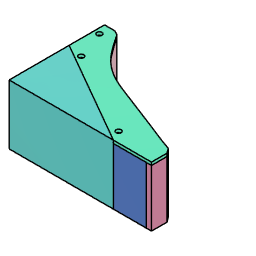
Version-1-reposabajo (Autodesk Fusion 360 archive; units mm, degrees)
design "Gomas bajo"
Autodesk Fusion 360 part; units mm, degrees
note: some values were not read from the file. Chosen so that the rebuilt part matches the saved one: which bodies a step acts on. Set by a fixed rule: which sketch regions a step uses.
sketch "Boceto1" plane through (0, 0, 0) normal (0, 1, 0) x (1, 0, 0)
  line L0 (0, 0) -> (381, 0)
  line L1 (0, 0) -> (0, 64.9)
  line L2 (381, 0) -> (381, 54.6)
  line L3 (381, 54.6) -> (327.1, 0)
  line L4 (0, 64.9) -> (168.7, 0)
  line L5 (0, 0) -> (0, 109.3)
  line L6 (0, 109.3) -> (62.7, 0)
  line L7 (168.7, 0) -> (168.7, 23.3)
  line L8 (168.7, 23.3) -> (326.4, 23.3)
  line L9 (326.4, 23.3) -> (326.4, 0)
  line L10 (0, 0) -> (0, -78.7)
  line L11 (0, -78.7) -> (-56.8, -78.7)
  line L12 (-56.8, -78.7) -> (-56.8, 0)
  line L13 (-56.8, 0) -> (0, 0)
  line L14 (0, 109.3) -> (168.7, 0)
  line L15 (32.6827, 52.3267) -> (381, 54.6)
  circle A0 centre (0, 64.9) radius 22.093
  line L16 (19.1638, 75.8933) -> (0, 64.9)
  arc A1 (19.1638, 75.8933) -> (58.0399, 42.5717) centre (85.4981, 113.946) ccw
  line L17 (104.1577, -30) -> (104.1577, 0)
  arc A2 (145.6154, 0) -> (62.7, 0) centre (104.1577, -30) ccw
  dimension "d1" = 381
  dimension "d2" = 64.9
  dimension "d3" = 54.6
  dimension "d4" = 53.9
  dimension "d5" = 168.7
  dimension "d6" = 109.3
  dimension "d7" = 62.7
  dimension "d8" = 23.3
  dimension "d9" = 157.7
  dimension "d10" = 78.7
  dimension "d11" = 56.8
  dimension "d14" = 30
  constraint coincident L0.start L1.start
  constraint horizontal L0
  constraint perpendicular L0 L1
  constraint perpendicular L0 L2
  constraint coincident L0 L3.end
  constraint coincident L0 L4.end
  constraint perpendicular L0 L5
  constraint coincident L0 L6.end
  constraint perpendicular L0 L7
  constraint perpendicular L7 L8
  constraint coincident L0 L9.end
  constraint perpendicular L0 L9
  constraint perpendicular L0 L10
  constraint perpendicular L10 L11
  constraint perpendicular L11 L12
  constraint perpendicular L10 L13
  constraint coincident L6 L15.start
  constraint coincident L4 L15.start
  constraint coincident L1.end L4.start
  constraint tangent L6 A0
  constraint tangent L6 A1
  constraint tangent L4 A1
  constraint coincident L6 L16.start
  constraint coincident A0 L16.start
  constraint perpendicular L6 L16
  constraint coincident L4 A1.end
  constraint tangent L4 A2
  constraint coincident L17.start A2.centre
  constraint coincident L0 L17.end
  constraint perpendicular L0 L17
  constraint coincident L0 A2.start
  measures "d1" distance of L0.start L0.end
  measures "d2" distance of L0.start L1.end
  measures "d3" distance of L0.end L2.end
  measures "d4" distance of L0.end L3.end
  measures "d5" distance of L0.start L4.end
  measures "d6" distance of L0.start L5.end
  measures "d7" distance of L0.start L6.end
  measures "d8" distance of L4.end L7.end
  measures "d9" distance of L7.end L8.end
  measures "d10" distance of L0.start L10.end
  measures "d11" distance of L10.end L11.end
  measures "d14" distance of L17.start L17.end
extrude "Extruir1" add sketch "Boceto1" along normal blind 120 contours L0 L1 L4 L5 L6 A0 | L10 L11 L12 L13 | L0 A2 | L4 L6 A2 | L1 L4 L5 A0 | L4 L15 A1 | L4 L6 A0 | L6 L15 A1 | L4 A0 L16 | L5 A0 L16 | L0 L7 L8 L9 | L0 L2 L3 makes body 3 at (48.5385, 80, 0) makes body 3 at (0, 40, 26.2333) makes body 2 at (363.0333, 40, -36.4) makes body 1 at (221.2667, 40, -23.3)
sketch "Boceto2" plane through (0, 120, 0) normal (0, 1, 0) x (-1, 0, 0)
  line L0 (0, 0) -> (-145.6154, 0)
  arc A0 (-145.6154, 0) -> (-122.5313, -17.7614) centre (-104.1577, 30) ccw
  line L1 (-122.5313, -17.7614) -> (-58.0399, -42.5717)
  arc A1 (-19.1638, -75.8933) -> (-58.0399, -42.5717) centre (-85.4981, -113.946) ccw
  arc A2 (-19.1638, -75.8933) -> (0, -86.993) centre (0, -64.9) ccw
  line L2 (0, -86.993) -> (0, 0)
  arc A3 (-137.514, 5.8624) -> (-118.9408, -8.4282) centre (-104.1577, 30) ccw
  line L3 (-118.9408, -8.4282) -> (-54.4494, -33.2385)
  arc A4 (-10.4896, -70.9174) -> (-54.4494, -33.2385) centre (-85.4981, -113.946) ccw
  arc A5 (-10.4896, -70.9174) -> (0, -76.993) centre (0, -64.9) ccw
  line L4 (-10, -84.6003) -> (-10, -10)
  line L5 (-10, -10) -> (-136.0754, -10)
  line L6 (-10.4896, -70.9174) -> (-85.4981, -113.946)
  line L7 (-85.4981, -113.946) -> (-54.4494, -33.2385)
  arc A6 (-143.9951, 1.1725) -> (-121.8132, -15.8948) centre (-104.1577, 30) ccw
  line L8 (-121.8132, -15.8948) -> (-57.3218, -40.705)
  arc A7 (-17.4289, -74.8981) -> (-57.3218, -40.705) centre (-85.4981, -113.946) ccw
  arc A8 (-17.4289, -74.8981) -> (0, -84.993) centre (0, -64.9) ccw
  arc A9 (-14.7871, -64.1697) -> (-4.4377, -76.1494) centre (-10.4896, -70.9174) ccw
  arc A10 (-24.2647, -52.887) -> (-14.0734, -65.1993) centre (-18.884, -58.8072) ccw
  arc A11 (-35.5202, -43.3773) -> (-23.3866, -53.7805) centre (-29.2125, -48.298) ccw
  arc A12 (-48.2269, -35.9166) -> (-34.5032, -44.1087) centre (-41.1754, -39.6949) ccw
  arc A13 (-61.8917, -30.3754) -> (-47.1004, -36.4648) centre (-54.4252, -33.2478) ccw
  arc A14 (-75.8914, -24.9896) -> (-60.9584, -30.7344) centre (-68.4249, -27.862) ccw
  arc A15 (-89.8912, -19.6038) -> (-74.9581, -25.3486) centre (-82.4247, -22.4762) ccw
  arc A16 (-103.891, -14.218) -> (-88.9579, -19.9628) centre (-96.4244, -17.0904) ccw
  arc A17 (-117.8907, -8.8322) -> (-102.9576, -14.577) centre (-110.4242, -11.7046) ccw
  arc A18 (-130.436, -1.6973) -> (-117.3466, -9.0415) centre (-124.4239, -6.3188) ccw
  arc A19 (-18.1953, -68.7673) -> (-19.5747, -66.7773) centre (-19.7105, -68.3445) ccw
  arc A20 (-26.8428, -57.9966) -> (-28.54, -56.2697) centre (-28.4078, -57.8372) ccw
  arc A21 (-37.1934, -48.8504) -> (-39.1592, -47.4367) centre (-38.7627, -48.959) ccw
  arc A22 (-48.9466, -41.5943) -> (-51.1238, -40.5349) centre (-50.4747, -41.9678) ccw
  arc A23 (-62.0016, -35.8165) -> (-64.5236, -34.8462) centre (-63.6663, -36.3809) ccw
  arc A24 (-76.0013, -30.4307) -> (-78.5233, -29.4604) centre (-77.6661, -30.9951) ccw
  arc A25 (-90.0011, -25.0449) -> (-92.5231, -24.0746) centre (-91.6658, -25.6093) ccw
  arc A26 (-104.0008, -19.6591) -> (-106.5228, -18.6888) centre (-105.6656, -20.2235) ccw
  arc A27 (-118.0703, -14.0576) -> (-120.7709, -12.9639) centre (-119.8658, -14.6102) ccw
  line L9 (-381, -54.6) -> (-327.1, 0)
  line L10 (-327.1, 0) -> (-381, 0)
  line L11 (-381, 0) -> (-381, -54.6)
  line L12 (-168.7, 0) -> (-326.4, 0)
  arc A28 (-288.7387, 0) -> (-354.05, -27.3) centre (-288.7387, -91.774) ccw
  line L13 (-354.05, -27.3) -> (-381, -54.6)
  arc A29 (-288.7387, 3) -> (-356.185, -25.1924) centre (-288.7387, -91.774) ccw
  line L14 (-356.185, -25.1924) -> (-383.135, -52.4924)
  arc A30 (-288.7387, 10) -> (-361.1665, -20.2747) centre (-288.7387, -91.774) ccw
  line L15 (-361.1665, -20.2747) -> (-388.1165, -47.5747)
  line L16 (-288.7387, -91.774) -> (-288.7387, 10)
  line L17 (-361.1665, -20.2747) -> (-288.7387, -91.774)
  arc A31 (-375.2171, -34.5078) -> (-365.3817, -24.5446) centre (-370.2994, -29.5262) ccw
  arc A32 (-381, -31.9555) -> (-374.5146, -33.7961) centre (-379.4323, -38.7777) ccw
  arc A33 (-366.0843, -25.2563) -> (-356.0804, -15.4652) centre (-361.1665, -20.2747) ccw
  arc A34 (-356.5009, -15.8383) -> (-345.4457, -7.2621) centre (-351.1209, -11.36) ccw
  arc A35 (-345.9117, -7.5766) -> (-333.8234, -0.5309) centre (-339.9888, -3.8458) ccw
  arc A36 (-334.3267, -0.7813) -> (-321.416, 4.6114) centre (-327.9641, 2.1372) ccw
  arc A37 (-330.9794, -4.1801) -> (-333.0783, -6.056) centre (-331.6366, -5.5569) ccw
  arc A38 (-342.146, -10.5051) -> (-344.138, -11.8497) centre (-342.6161, -11.9565) ccw
  arc A39 (-352.3824, -18.2454) -> (-354.18, -19.8407) centre (-352.6573, -19.7461) ccw
  arc A40 (-361.7084, -27.2537) -> (-363.328, -28.8943) centre (-361.8252, -28.7581) ccw
  arc A41 (-370.8413, -36.5052) -> (-372.4609, -38.1458) centre (-370.9581, -38.0096) ccw
  line L18 (-332.7328, 0) -> (-321.2984, 0)
  arc A42 (-133.4633, 8.7936) -> (-117.1456, -3.7616) centre (-104.1577, 30) ccw
  line L19 (-117.1456, -3.7616) -> (-52.6541, -28.5719)
  arc A43 (-6.1526, -68.4294) -> (-52.6541, -28.5719) centre (-85.4981, -113.946) ccw
  arc A44 (-6.1526, -68.4294) -> (0, -71.993) centre (0, -64.9) ccw
  line L20 (-321.2984, 0) -> (-321.2984, 10)
  line L21 (-341, 10) -> (-321.2984, 10)
  line L22 (-341, 10) -> (-381, -30)
  line L23 (-381, 0) -> (-386, 0)
  line L24 (-386, 0) -> (-386, -54.6)
  line L25 (-386, -54.6) -> (-381, -54.6)
  point P0 (-10.4896, -70.9174)
  point P1 (-18.884, -58.8072)
  point P2 (-29.2125, -48.298)
  point P3 (-41.1754, -39.6949)
  point P4 (-54.4252, -33.2478)
  point P5 (-68.4249, -27.862)
  point P6 (-82.4247, -22.4762)
  point P7 (-96.4244, -17.0904)
  point P8 (-110.4242, -11.7046)
  point P9 (-124.4239, -6.3188)
  point P10 (-351.1209, -11.36)
  point P11 (-339.9888, -3.8458)
  point P12 (-327.9641, 2.1372)
  point P13 (-315.2564, 6.4846)
  point P14 (-302.0868, 9.1209)
  point P15 (-288.6848, 10)
  point P16 (-370.2994, -29.5262)
  point P17 (-379.4323, -38.7777)
  dimension "d15" = -10
  dimension "d19" = 39.117
  dimension "d21" = 39.1
  dimension "d24" = -15
  dimension "d25" = 0
  dimension "d26" = -2
  dimension "d27" = 3
  dimension "d28" = 10
  dimension "d30" = -45.4
  dimension "d33" = 13
  dimension "d34" = 0
  dimension "d37" = -15
  dimension "d38" = 10
  dimension "d39" = 45
  dimension "d40" = 30
  dimension "d41" = 5
  constraint coincident A2 L4.start
  constraint coincident A0 L5.end
  constraint coincident P0 A4.start
  constraint coincident A1.centre A4.centre
  constraint coincident A7.start A9
  constraint coincident P1 A10.centre
  constraint tangent A7 A10
  constraint coincident P2 A11.centre
  constraint tangent A7 A11
  constraint coincident P3 A12.centre
  constraint tangent A7 A12
  constraint coincident P4 A13.centre
  constraint coincident L8.end A13
  constraint coincident P5 A14.centre
  constraint tangent L8 A14
  constraint coincident P6 A15.centre
  constraint tangent L8 A15
  constraint coincident P7 A16.centre
  constraint tangent L8 A16
  constraint coincident P8 A17.centre
  constraint tangent L8 A17
  constraint coincident P9 A18.centre
  constraint tangent A6 A18
  constraint coincident A5 A9.end
  constraint coincident A4 A10.end
  constraint coincident A4 A9.start
  constraint coincident A4 A10.start
  constraint coincident A4 A11.end
  constraint coincident A4 A12.end
  constraint coincident A4 A11.start
  constraint coincident A4 A12.start
  constraint coincident A4 A13.end
  constraint coincident L3 A14.end
  constraint coincident L3 A13.start
  constraint coincident L3 A15.end
  constraint coincident L3 A14.start
  constraint coincident L3 A15.start
  constraint coincident L3 A16.end
  constraint coincident L3 A17.end
  constraint coincident L3 A16.start
  constraint coincident L3 A18.end
  constraint coincident L3 A17.start
  constraint coincident A3 A18.start
  constraint tangent A7 A19
  constraint tangent A10 A19
  constraint tangent A9 A19
  constraint tangent A10 A20
  constraint tangent A11 A20
  constraint tangent A7 A20
  constraint tangent A7 A21
  constraint tangent A11 A21
  constraint tangent A12 A21
  constraint tangent A7 A22
  constraint tangent A13 A22
  constraint tangent A12 A22
  constraint tangent L8 A23
  constraint tangent A13 A23
  constraint tangent A14 A23
  constraint tangent A14 A24
  constraint tangent L8 A24
  constraint tangent A15 A24
  constraint tangent A15 A25
  constraint tangent L8 A25
  constraint tangent A16 A25
  constraint tangent A16 A26
  constraint tangent A17 A26
  constraint tangent L8 A26
  constraint tangent A17 A27
  constraint tangent A18 A27
  constraint tangent A6 A27
  constraint coincident A9 A19.start
  constraint coincident A10 A19.end
  constraint coincident A10 A20.start
  constraint coincident A11 A20.end
  constraint coincident A11 A21.start
  constraint coincident A12 A21.end
  constraint coincident A13 A22.end
  constraint coincident A12 A22.start
  constraint coincident A13 A23.start
  constraint coincident A14 A23.end
  constraint coincident A14 A24.start
  constraint coincident A15 A24.end
  constraint coincident A15 A25.start
  constraint coincident A16 A25.end
  constraint coincident A16 A26.start
  constraint coincident A17 A26.end
  constraint coincident A18 A27.end
  constraint coincident A17 A27.start
  constraint tangent L9 A28
  constraint tangent L12 A28
  constraint midpoint L9 A28.end
  constraint coincident L12 A28.start
  constraint coincident L9.start L11.end
  constraint coincident A28.centre A29.centre
  constraint perpendicular L12 L16
  constraint coincident P12 A36.centre
  constraint coincident P11 A35.centre
  constraint coincident P10 A34.centre
  constraint coincident A30.end L15.start
  constraint coincident P16 A31.centre
  constraint coincident P17 A32.centre
  constraint tangent A29 A36
  constraint tangent A29 A35
  constraint tangent A29 A34
  constraint tangent A29 A33
  constraint tangent L14 A31
  constraint tangent L14 A32
  constraint tangent A36 A37
  constraint tangent A35 A37
  constraint tangent A29 A37
  constraint tangent A34 A38
  constraint tangent A35 A38
  constraint tangent A29 A38
  constraint tangent A29 A39
  constraint tangent A34 A39
  constraint tangent A33 A39
  constraint tangent L14 A40
  constraint tangent A33 A40
  constraint tangent A31 A40
  constraint tangent L14 A41
  constraint tangent A31 A41
  constraint tangent A32 A41
  constraint coincident L15 A31.start
  constraint coincident L15 A32.end
  constraint coincident L11 A32.start
  constraint coincident L15 A33.start
  constraint coincident L15 A31.end
  constraint coincident A30 A34.start
  constraint coincident A30 A33.end
  constraint coincident A30 A35.start
  constraint coincident A30 A34.end
  constraint coincident A30 A36.end
  constraint coincident A30 A36.start
  constraint coincident A30 A35.end
  constraint coincident A36 A37.start
  constraint coincident L9 A37.end
  constraint coincident A35 A38.start
  constraint coincident A34 A38.end
  constraint coincident A34 A39.start
  constraint coincident A33 A39.end
  constraint coincident A33 A40.start
  constraint coincident A31 A40.end
  constraint coincident A31 A41.start
  constraint coincident A32 A41.end
  constraint coincident A30 L18.start
  constraint coincident L10 L18.start
  constraint coincident A36 L18.end
  constraint coincident L12 L18.end
  constraint perpendicular L10 L20
  constraint perpendicular L20 L21
  constraint coincident L11 L22.end
  constraint coincident L10.end L11.start
  constraint perpendicular L11 L23
  constraint perpendicular L23 L24
  constraint perpendicular L11 L25
  measures "d19" angle of L6 L7
  measures "d38" distance of L18.end L20.end
  measures "d39" angle of L21 L22
  measures "d40" distance of L10.end L22.end
  measures "d41" distance of L10.end L23.end
extrude "Extruir2" add sketch "Boceto2" against normal blind 110 separate body contours L3 A4 A5 L4 L5 L19 A43 | L5 A6 A18 | L5 A17 A18 | L3 L5 A16 A17 A18 | L4 A8 A9 | A5 L4 L6 A9 | L5 A17 A18 | L3 A16 A17 | A4 L6 A9 A10 | A4 L7 A12 A13 | A17 A18 A27 | L3 A15 A16 A17 | A16 A17 A26 | A4 A9 A10 A11 | A9 A10 A19 | A4 A9 A10 | L3 A15 A16 | A4 A10 A11 A12 | A10 A11 A20 | L3 L7 A13 A14 | L3 A14 A15 A16 | A15 A16 A25 | A4 A11 A12 A13 | A11 A12 A21 | A4 A10 A11 | L3 A13 A14 A15 | A13 A14 A23 | A12 A13 A22 | L3 A14 A15 | A4 A11 A12 | L3 A13 A14 | A4 A12 A13 | A14 A15 A24 | L11 L14 A32 | L15 L17 A31 A33 | A30 L17 A33 A34 | L11 L15 A31 A32 | L9 A30 A34 A35 A36 | L9 A35 | A30 A33 A34 A35 | L15 A31 A32 A33 | L10 L11 A30 L15 L22 | A31 A33 A40 | A33 A34 A39 | A31 A32 A41 | A34 A35 A38 | L9 L12 A36 L18 | L10 L12 A30 A36 L18 L20 | A30 A33 A34 | L15 A31 A33 | L15 A31 A32 | L9 A35 A36 A37 | A30 A34 A35 | L10 A30 L20 L21 L22 | A30 A35 A36 | L9 L10 A30 A35 A36 L18 makes body 4 at (12.1388, 46.6667, -59.3028) makes body 5 at (354.3333, 83.3333, -3.3333)
copy_body "Cuerpo - > Comp.1" bodies 4 removing the originals makes body 6 in component "GOMAS"
copy_body "Cuerpo - > Comp.2" bodies 5 removing the originals makes body 7 in component "GOMA AUXILIAR"
sketch "Boceto6" plane through (0, 120, 0) normal (0, 1, 0) x (-1, 0, 0)
  arc A0 (-18.1953, -68.7673) -> (-17.4289, -74.8981) centre (-10.4896, -70.9174) ccw
  arc A1 (-17.4289, -74.8981) -> (-10, -82.3279) centre (0, -64.9) ccw
  line L0 (-10, -82.3279) -> (-10, -62.2981)
  arc A2 (-10, -62.2981) -> (-52.6541, -28.5719) centre (-85.4981, -113.946) ccw
  line L1 (-52.6541, -28.5719) -> (-100.9296, -10)
  line L2 (-100.9296, -10) -> (-132.7592, -10)
  arc A3 (-132.7592, -10) -> (-128.119, -12.9407) centre (-104.1577, 30) ccw
  arc A4 (-128.119, -12.9407) -> (-120.7709, -12.9639) centre (-124.4239, -6.3188) ccw
  arc A5 (-118.0703, -14.0576) -> (-120.7709, -12.9639) centre (-119.8658, -14.6102) ccw
  arc A6 (-118.0703, -14.0576) -> (-106.5228, -18.6888) centre (-110.4242, -11.7046) ccw
  arc A7 (-104.0008, -19.6591) -> (-106.5228, -18.6888) centre (-105.6656, -20.2235) ccw
  arc A8 (-104.0008, -19.6591) -> (-92.5231, -24.0746) centre (-96.4244, -17.0904) ccw
  arc A9 (-90.0011, -25.0449) -> (-92.5231, -24.0746) centre (-91.6658, -25.6093) ccw
  arc A10 (-90.0011, -25.0449) -> (-78.5233, -29.4604) centre (-82.4247, -22.4762) ccw
  arc A11 (-76.0013, -30.4307) -> (-78.5233, -29.4604) centre (-77.6661, -30.9951) ccw
  arc A12 (-76.0013, -30.4307) -> (-64.5236, -34.8462) centre (-68.4249, -27.862) ccw
  arc A13 (-62.0016, -35.8165) -> (-64.5236, -34.8462) centre (-63.6663, -36.3809) ccw
  arc A14 (-62.0016, -35.8165) -> (-57.3218, -40.705) centre (-54.4252, -33.2478) ccw
  arc A15 (-57.2779, -40.7219) -> (-57.3218, -40.705) centre (-85.4981, -113.946) ccw
  arc A16 (-57.2779, -40.7219) -> (-51.1238, -40.5349) centre (-54.4252, -33.2478) ccw
  arc A17 (-48.9466, -41.5943) -> (-51.1238, -40.5349) centre (-50.4747, -41.9678) ccw
  arc A18 (-48.9466, -41.5943) -> (-39.1592, -47.4367) centre (-41.1754, -39.6949) ccw
  arc A19 (-37.1934, -48.8504) -> (-39.1592, -47.4367) centre (-38.7627, -48.959) ccw
  arc A20 (-37.1934, -48.8504) -> (-28.54, -56.2697) centre (-29.2125, -48.298) ccw
  arc A21 (-26.8428, -57.9966) -> (-28.54, -56.2697) centre (-28.4078, -57.8372) ccw
  arc A22 (-26.8428, -57.9966) -> (-19.5747, -66.7773) centre (-18.884, -58.8072) ccw
  arc A23 (-18.1953, -68.7673) -> (-19.5747, -66.7773) centre (-19.7105, -68.3445) ccw
  line L3 (-10, -62.2981) -> (-10, -47.2981)
  line L4 (-100.9296, -10) -> (-100.9296, 5)
  line L5 (-10, -47.2981) -> (-100.9296, 5)
  line L6 (-132.7592, -10) -> (-132.7592, 5)
  line L7 (-132.7592, 5) -> (-100.9296, 5)
  circle A24 centre (-95.9296, -5) radius 2.5
  circle A25 centre (-15, -49.7981) radius 2.5
  line L8 (-10, -82.3279) -> (0, -82.3279)
  line L9 (0, -82.3279) -> (0, -53.0496)
  line L10 (-10, -47.2981) -> (0, -53.0496)
  circle A26 centre (-5, -77.3279) radius 2.5
  line L11 (0, -82.3279) -> (0, -87.3279)
  spline S0 degree 5 poles (-10, -82.3279) (-10.3791, -81.7612) (-11.1335, -80.6369) (-12.2536, -78.9772) (-13.7241, -76.818) (-15.5252, -74.2085) (-17.2927, -71.6878) (-19.0339, -69.2548) (-20.7609, -66.9069) (-22.4923, -64.6401) (-24.2517, -62.4495) (-26.063, -60.3298) (-27.9469, -58.2772) (-29.9176, -56.2895) (-31.9775, -54.3677) (-34.1205, -52.5154) (-36.3353, -50.7374) (-38.6098, -49.039) (-40.9343, -47.4243) (-43.306, -45.8961) (-45.7265, -44.4546) (-48.1994, -43.0976) (-50.7279, -41.8197) (-53.3125, -40.6122) (-55.9486, -39.4627) (-58.6283, -38.3568) (-61.342, -37.2799) (-64.0798, -36.2183) (-66.8331, -35.1616) (-69.5958, -34.1035) (-72.3637, -33.0409) (-75.134, -31.9736) (-77.9049, -30.903) (-80.6749, -29.8316) (-83.4425, -28.7623) (-86.2064, -27.6977) (-88.9661, -26.6393) (-91.7219, -25.5871) (-94.4755, -24.539) (-97.2302, -23.4898) (-99.9899, -22.4333) (-102.7578, -21.3638) (-105.5358, -20.2776) (-108.323, -19.1752) (-111.115, -18.0622) (-113.9047, -16.9486) (-116.6836, -15.8463) (-119.4432, -14.7673) (-122.1762, -13.7225) (-124.8773, -12.7189) (-127.5439, -11.7608) (-129.6482, -11.0324) (-131.2101, -10.5078) (-132.2441, -10.1677) (-132.7592, -10) knots 0 0 0 0 0 0 0.02 0.04 0.06 0.08 0.1 0.12 0.14 0.16 0.18 0.2 0.22 0.24 0.26 0.28 0.3 0.32 0.34 0.36 0.38 0.4 0.42 0.44 0.46 0.48 0.5 0.52 0.54 0.56 0.58 0.6 0.62 0.64 0.66 0.68 0.7 0.72 0.74 0.76 0.78 0.8 0.82 0.84 0.86 0.88 0.9 0.92 0.94 0.96 0.98 1 1 1 1 1 1
  spline S1 degree 3 poles (-14.1557, -85.1082) (-17.5783, -79.9925) (-20.7861, -75.3183) (-23.853, -71.151) (-26.9809, -66.9009) (-29.9853, -63.2205) (-33.4712, -59.8464) (-37.018, -56.4134) (-41.0443, -53.2779) (-45.2613, -50.6011) (-49.2492, -48.0696) (-53.4516, -45.9665) (-58.0406, -44.0221) (-62.9252, -41.9524) (-68.1989, -39.997) (-73.4701, -37.9714) (-79.5139, -35.6489) (-85.555, -33.2968) (-91.5498, -31.0055) (-96.5278, -29.1028) (-101.5185, -27.22) (-106.5821, -25.2352) (-112.5778, -22.8851) (-118.611, -20.4076) (-124.3266, -18.263) (-127.7512, -16.9779) (-131.0771, -15.8056) (-134.3066, -14.7545) knots 0 0 0 0 0.109182 0.109182 0.109182 0.220535 0.220535 0.220535 0.333833 0.333833 0.333833 0.440981 0.440981 0.440981 0.555032 0.555032 0.555032 0.685799 0.685799 0.685799 0.794386 0.794386 0.794386 0.92296 0.92296 0.92296 1 1 1 1
  line L12 (-132.7592, 5) -> (-137.7592, 5)
  line L13 (-137.7592, 5) -> (-137.7592, -10)
  line L14 (-137.7592, -10) -> (-132.7592, -10)
  line L15 (-137.7592, -10) -> (-134.3066, -14.7545)
  line L16 (-10, -82.3279) -> (-10, -87.3279)
  line L17 (-10, -87.3279) -> (0, -87.3279)
  line L18 (-14.1557, -85.1082) -> (-10, -87.3279)
  point P0 (-19.7105, -68.3445)
  point P1 (-28.4078, -57.8372)
  point P2 (-38.7627, -48.959)
  point P3 (-50.4747, -41.9678)
  point P4 (-63.6663, -36.3809)
  point P5 (-77.6661, -30.9951)
  point P6 (-91.6658, -25.6093)
  point P7 (-105.6656, -20.2235)
  point P8 (-119.8658, -14.6102)
  dimension "d42" = 15
  dimension "d43" = 15
  dimension "d44" = 15
  dimension "d45" = 5
  dimension "d46" = 5
  dimension "d47" = 5
  dimension "d48" = 2.5
  dimension "d49" = 5
  dimension "d50" = 5
  dimension "d75" = 10
  dimension "d76" = 5
  dimension "d77" = 5
  dimension "d78" = 5
  dimension "d83" = 5
  dimension "d84" = -5
  dimension "d85" = 5
  dimension "d86" = 15
  dimension "d87" = 5
  constraint coincident L0.end A2.start
  constraint parallel L0 L3
  constraint coincident L1.end L2.start
  constraint perpendicular L2 L4
  constraint coincident L2.end A3.start
  constraint perpendicular L2 L6
  constraint coincident A1.end L0.start
  constraint perpendicular L3 L8
  constraint perpendicular L8 L9
  constraint parallel L5 L10
  constraint coincident L9.end L10.end
  constraint perpendicular L8 L11
  constraint coincident P0 A23.centre
  constraint coincident P1 A21.centre
  constraint coincident P2 A19.centre
  constraint coincident P3 A17.centre
  constraint coincident P4 A13.centre
  constraint coincident P5 A11.centre
  constraint coincident P6 A9.centre
  constraint coincident P7 A7.centre
  constraint coincident P8 A5.centre
  constraint perpendicular L6 L12
  constraint perpendicular L12 L13
  constraint perpendicular L8 L16
  measures "d42" distance of L0.end L3.end
  measures "d43" distance of L1.end L4.end
  measures "d44" distance of L2.end L6.end
  measures "d45" diameter of A24
  measures "d46" diameter of A25
  measures "d47" distance of L3 A25.centre
  measures "d48" vertical distance of L3.end A25.centre
  measures "d49" distance of L4 A24.centre
  measures "d50" vertical distance of L1.end A24.centre
  measures "d75" distance of A1.end L8.end
  measures "d76" diameter of A26
  measures "d77" distance of L9 A26.centre
  measures "d78" distance of L8 A26.centre
  measures "d83" distance of L8.end L11.end
  measures "d85" distance of L6.end L12.end
  measures "d86" distance of L12.end L13.end
  measures "d87" distance of A1.end L16.end
extrude "Extruir1'" add sketch "Boceto6" against normal blind 110 separate body contours L0 L3 L8 L9 L10 | A2 L1 L3 L4 L5 | L2 L4 L6 L7 makes body 8 in component "BASES"
sketch "Boceto1 (2)" plane through (10, 0, 0) normal (-1, 0, 0) x (0, 0, 1) in component "GOMAS"
  line L0 (-62.2981, 120) -> (-82.3279, 120)
  line L1 (-82.3279, 120) -> (-82.3279, 10)
  line L2 (-82.3279, 10) -> (-62.2981, 10)
  line L3 (-62.2981, 10) -> (-62.2981, 120)
  line L4 (-62.2981, 65) -> (-82.3279, 65)
  line L5 (-72.313, 120) -> (-72.313, 10)
  line L6 (-72.313, 100) -> (-77.313, 100)
  line L7 (-77.313, 100) -> (-77.313, 75)
  line L8 (-77.313, 75) -> (-67.313, 75)
  line L9 (-67.313, 75) -> (-67.313, 80)
  line L10 (-67.313, 80) -> (-72.313, 80)
  line L11 (-72.313, 100) -> (-67.313, 100)
  line L12 (-67.313, 100) -> (-67.313, 95)
  line L13 (-67.313, 95) -> (-72.313, 95)
  line L14 (-67.313, 30) -> (-67.313, 35)
  line L15 (-67.313, 50) -> (-72.313, 50)
  line L16 (-72.313, 30) -> (-77.313, 30)
  line L17 (-67.313, 35) -> (-72.313, 35)
  line L18 (-72.313, 30) -> (-67.313, 30)
  line L19 (-77.313, 30) -> (-77.313, 55)
  line L20 (-67.313, 55) -> (-67.313, 50)
  line L21 (-77.313, 55) -> (-67.313, 55)
  dimension "d57" = 5
  dimension "d58" = 25
  dimension "d59" = 10
  dimension "d60" = 5
  dimension "d61" = 5
  dimension "d62" = 10
  dimension "d63" = 5
  constraint midpoint L3 L4.start
  constraint midpoint L1 L4.end
  constraint midpoint L0 L5.start
  constraint midpoint L2 L5.end
  constraint coincident L5 L6.start
  constraint perpendicular L5 L6
  constraint perpendicular L6 L7
  constraint perpendicular L5 L8
  constraint perpendicular L8 L9
  constraint coincident L5 L10.end
  constraint perpendicular L5 L10
  constraint perpendicular L5 L11
  constraint perpendicular L11 L12
  constraint coincident L5 L13.end
  constraint perpendicular L5 L13
  constraint symmetric L4 L6.start L16.start
  constraint symmetric L4 L6.end L16.end
  constraint symmetric L4 L7.end L19.end
  constraint symmetric L4 L8.end L20.start
  constraint symmetric L4 L9.end L15.start
  constraint symmetric L4 L10.end L15.end
  constraint symmetric L4 L11.end L14.start
  constraint symmetric L4 L12.end L14.end
  constraint symmetric L4 L13.end L17.end
  measures "d57" distance of L6.start L6.end
  measures "d58" distance of L6.end L7.end
  measures "d59" distance of L7.end L8.end
  measures "d60" distance of L8.end L9.end
  measures "d61" distance of L11.end L12.end
  measures "d62" distance of L4 L7.end
  measures "d63" distance of L6.start L11.end
extrude "Extruir1''" cut sketch "Boceto1 (2)" against normal blind 2 contours L5 L11 L12 L13 | L5 L6 L7 L8 | L5 L8 L9 L10 | L5 L15 L20 L21 | L5 L16 L19 L21 | L5 L14 L17 L18 bodies 6 in component "GOMAS"
sketch "Boceto2 (2)" plane through (0, 0, -10) normal (0, 0, 1) x (1, 0, 0) in component "GOMAS"
  line L0 (132.7592, 120) -> (100.9296, 120)
  line L1 (100.9296, 120) -> (100.9296, 10)
  line L2 (100.9296, 10) -> (132.7592, 10)
  line L3 (132.7592, 10) -> (132.7592, 120)
  line L4 (116.8444, 120) -> (116.8444, 10)
  line L5 (100.9296, 65) -> (132.7592, 65)
  line L6 (106.8444, 100) -> (116.8444, 100)
  line L7 (116.8444, 100) -> (116.8444, 75)
  line L8 (116.8444, 75) -> (106.8444, 75)
  line L9 (106.8444, 75) -> (106.8444, 80)
  line L10 (106.8444, 80) -> (111.8444, 80)
  line L11 (111.8444, 80) -> (111.8444, 95)
  line L12 (111.8444, 95) -> (106.8444, 95)
  line L13 (106.8444, 95) -> (106.8444, 100)
  line L14 (111.8444, 35) -> (106.8444, 35)
  line L15 (116.8444, 30) -> (116.8444, 55)
  line L16 (106.8444, 55) -> (106.8444, 50)
  line L17 (106.8444, 35) -> (106.8444, 30)
  line L18 (106.8444, 50) -> (111.8444, 50)
  line L19 (116.8444, 55) -> (106.8444, 55)
  line L20 (111.8444, 50) -> (111.8444, 35)
  line L21 (106.8444, 30) -> (116.8444, 30)
  dimension "d66" = 10
  dimension "d67" = 25
  dimension "d68" = 10
  dimension "d69" = 5
  dimension "d70" = 5
  dimension "d71" = 15
  dimension "d72" = 10
  constraint midpoint L0 L4.start
  constraint midpoint L2 L4.end
  constraint midpoint L1 L5.start
  constraint midpoint L3 L5.end
  constraint perpendicular L4 L6
  constraint perpendicular L6 L7
  constraint perpendicular L4 L8
  constraint perpendicular L6 L9
  constraint perpendicular L9 L10
  constraint perpendicular L10 L11
  constraint perpendicular L11 L12
  constraint perpendicular L6 L13
  constraint coincident L4 L7.end
  constraint symmetric L5 L6.start L17.end
  constraint symmetric L5 L6.end L15.start
  constraint symmetric L5 L7.end L15.end
  constraint symmetric L5 L8.end L16.start
  constraint symmetric L5 L9.end L16.end
  constraint symmetric L5 L10.end L18.end
  constraint symmetric L5 L11.end L14.start
  constraint symmetric L5 L12.end L14.end
  measures "d66" distance of L6.start L6.end
  measures "d67" distance of L6.end L7.end
  measures "d68" distance of L7.end L8.end
  measures "d69" distance of L8.end L9.end
  measures "d70" distance of L9.end L10.end
  measures "d71" distance of L10.end L11.end
  measures "d72" distance of L5 L7.end
extrude "Extruir2'" cut sketch "Boceto2 (2)" against normal blind 2 contours L4 L6 L7 L8 L9 L10 L11 L12 L13 | L4 L14 L15 L16 L17 L18 L19 L20 L21 bodies 6 in component "GOMAS"
split "Dividir1" by curves path "Boceto1 (2)" along L4 bodies 6 makes body 9 at (12.1388, 83.3333, -59.3028) in component "GOMAS"
copy_body "Cuerpo - > Comp.1'" bodies 6 removing the originals makes body 10 in component "GOMA 1"
copy_body "Cuerpo - > Comp.2'" bodies 9 removing the originals makes body 11 in component "Component"
ref_plane "PlanoDeObra1" through (66.3796, 65, -38.6639) normal (0, 1, 0) x (-1, 0, 0) in component "BASES"
split "Dividir1'" by plane through (66.3796, 65, -38.6639) normal (0, 1, 0) bodies 8 makes body 12 at (40.3099, 101.6667, -29.8654) in component "BASES"
copy_body "Cuerpo - > Comp.1''" bodies 8 removing the originals makes body 13 in component "BASE 1"
copy_body "Cuerpo - > Comp.2''" bodies 12 removing the originals makes body 14 in component "Component'"
extrude "Extruir1'''" add 1 faces at (12, 40, -75.6463) along direction (-1, 0, 0) blind 2 on bodies 10 bodies 13 in component "BASE 1"
extrude "Extruir2''" add 1 faces at (115.1777, 45, -12) along direction (0, 0, 1) blind 2 on bodies 10 bodies 13 in component "BASE 1"
extrude "Extruir1''''" add sketch "Boceto6" against normal blind 110 separate body contours A0 A22 A23 S0 | A0 A1 A3 A4 A6 A8 A10 A12 A14 A15 A16 A18 A20 A22 S0 S1 L14 L15 L16 L18 | L8 L11 L16 L17 | A20 A21 A22 S0 | A18 A19 A20 S0 | L6 L12 L13 L14 | A4 A5 A6 S0 | A16 A17 A18 S0 | A6 A7 A8 S0 | A12 A13 A14 S0 | A8 A9 A10 S0 | A10 A11 A12 S0 makes body 15 in component "TAPA"
split "Dividir1''" by plane through (66.3796, 65, -38.6639) normal (0, 1, 0) bodies 15 makes body 16 at (99.2115, 83.3333, -28.0832) in component "TAPA"
copy_body "Cuerpo - > Comp.1'''" bodies 15 removing the originals makes body 17 in component "TAPA 1"
copy_body "Cuerpo - > Comp.2'''" bodies 16 removing the originals makes body 18 in component "Component''"
extrude "Extruir2'''" add sketch "Boceto6" along normal blind 2.8 separate body makes body 19 in component "BASES"
copy_body "Cuerpo - > Comp.3" bodies 19 removing the originals makes body 20 in component "TAPA INFERIOR"
sketch "Boceto7" plane through (0, 10, 0) normal (0, -1, 0) x (1, 0, 0)
  arc A0 (17.4289, -74.8981) -> (18.1953, -68.7673) centre (10.4896, -70.9174) ccw
  arc A1 (19.5747, -66.7773) -> (18.1953, -68.7673) centre (19.7105, -68.3445) ccw
  arc A2 (19.5747, -66.7773) -> (26.8428, -57.9966) centre (18.884, -58.8072) ccw
  arc A3 (28.54, -56.2697) -> (26.8428, -57.9966) centre (28.4078, -57.8372) ccw
  arc A4 (28.54, -56.2697) -> (37.1934, -48.8504) centre (29.2125, -48.298) ccw
  arc A5 (39.1592, -47.4367) -> (37.1934, -48.8504) centre (38.7627, -48.959) ccw
  arc A6 (39.1592, -47.4367) -> (48.9466, -41.5943) centre (41.1754, -39.6949) ccw
  arc A7 (51.1238, -40.5349) -> (48.9466, -41.5943) centre (50.4747, -41.9678) ccw
  arc A8 (51.1238, -40.5349) -> (57.2779, -40.7219) centre (54.4252, -33.2478) ccw
  arc A9 (57.3218, -40.705) -> (57.2779, -40.7219) centre (85.4981, -113.946) ccw
  arc A10 (57.3218, -40.705) -> (62.0016, -35.8165) centre (54.4252, -33.2478) ccw
  arc A11 (64.5236, -34.8462) -> (62.0016, -35.8165) centre (63.6663, -36.3809) ccw
  arc A12 (64.5236, -34.8462) -> (76.0013, -30.4307) centre (68.4249, -27.862) ccw
  arc A13 (78.5233, -29.4604) -> (76.0013, -30.4307) centre (77.6661, -30.9951) ccw
  arc A14 (78.5233, -29.4604) -> (90.0011, -25.0449) centre (82.4247, -22.4762) ccw
  arc A15 (92.5231, -24.0746) -> (90.0011, -25.0449) centre (91.6658, -25.6093) ccw
  arc A16 (92.5231, -24.0746) -> (104.0008, -19.6591) centre (96.4244, -17.0904) ccw
  arc A17 (106.5228, -18.6888) -> (104.0008, -19.6591) centre (105.6656, -20.2235) ccw
  arc A18 (106.5228, -18.6888) -> (118.0703, -14.0576) centre (110.4242, -11.7046) ccw
  arc A19 (120.7709, -12.9639) -> (118.0703, -14.0576) centre (119.8658, -14.6102) ccw
  arc A20 (120.7709, -12.9639) -> (128.119, -12.9407) centre (124.4239, -6.3188) ccw
  arc A21 (128.119, -12.9407) -> (132.7592, -10) centre (104.1577, 30) ccw
  line L0 (132.7592, -10) -> (100.9296, -10)
  line L1 (100.9296, -10) -> (52.6541, -28.5719)
  arc A22 (52.6541, -28.5719) -> (10, -62.2981) centre (85.4981, -113.946) ccw
  line L2 (10, -62.2981) -> (10, -82.3279)
  arc A23 (10, -82.3279) -> (17.4289, -74.8981) centre (0, -64.9) ccw
  circle A24 centre (95.9296, -5) radius 2.5
  line L3 (132.7592, -10) -> (132.7592, 5)
  line L4 (0, -82.3279) -> (0, -53.0496)
  line L5 (0, -53.0496) -> (0, 5)
  circle A25 centre (15, -49.7981) radius 2.5
  circle A26 centre (95.9296, -5) radius 2.5
  circle A27 centre (5, -77.3279) radius 2.5
  line L6 (0, -82.3279) -> (10, -82.3279)
  line L7 (10, -82.3279) -> (10, -62.2981)
  arc A28 (52.6541, -28.5719) -> (10, -62.2981) centre (85.4981, -113.946) ccw
  line L8 (52.6541, -28.5719) -> (100.9296, -10)
  line L9 (100.9296, -10) -> (132.7592, -10)
  line L10 (132.7592, -10) -> (132.7592, 5)
  line L11 (132.7592, 5) -> (100.9296, 5)
  line L12 (100.9296, 5) -> (0, -53.0496)
  line L13 (0, -53.0496) -> (0, -82.3279)
  line L14 (100.9296, 5) -> (0, 5)
  point P0 (132.7592, -10)
  point P1 (10, -82.3279)
  dimension "d102" = 122.7592
  dimension "d103" = 72.3279
  dimension "d104" = 100.9296
  dimension "d105" = 58.0496
  constraint coincident L4.end L5.start
  constraint parallel L4 L5
  constraint coincident L11.end L12.start
  constraint perpendicular L5 L14
  constraint coincident L5.end L14.end
  measures "d102" distance of L2 L3
  measures "d103" vertical distance of P0 P1
  measures "d104" distance of L11.end L5.end
  measures "d105" distance of L4.end L5.end
extrude "Extruir1'''''" add sketch "Boceto7" against normal blind 57.8 separate body contours L5 L12 L14 makes body 21 in component "BASE MADERA INFERIOR"
extrude "Extruir1''''''" [suppressed] in component "Pestaña"
component "GOMA AUXILIAR" placed x (1, 0, 0) y (0, 1, 0) z (0, 0, 1) at (-190, 0, 50)
component "GOMAS" placed x (1, 0, 0) y (0, 1, 0) z (0, 0, 1) at (0, 0, 0)
component "BASES" placed x (1, 0, 0) y (0, 1, 0) z (0, 0, 1) at (0, 0, 0)
component "GOMA 1" placed x (1, 0, 0) y (0, 1, 0) z (0, 0, 1) at (0, 0, 0) in component "GOMAS"
component "Component" placed x (1, 0, 0) y (0, 1, 0) z (0, 0, 1) at (0, 0, 0) in component "GOMAS"
component "TAPA" placed x (1, 0, 0) y (0, 1, 0) z (0, 0, 1) at (0, 0, 0) in component "BASES"
component "Component'" placed x (1, 0, 0) y (0, 1, 0) z (0, 0, 1) at (0, 0, 0) in component "BASES"
component "BASE 1" placed x (1, 0, 0) y (0, 1, 0) z (0, 0, 1) at (0, 0, 0) in component "BASES"
component "TAPA INFERIOR" placed x (1, 0, 0) y (0, 1, 0) z (0, 0, 1) at (0, -55, 0) in component "BASES"
component "BASE MADERA INFERIOR" placed x (1, 0, 0) y (0, 1, 0) z (0, 0, 1) at (0, 0, 0) in component "BASES"
component "Component''" placed x (1, 0, 0) y (0, 1, 0) z (0, 0, 1) at (0, 0, 0) in component "TAPA"
component "TAPA 1" placed x (1, 0, 0) y (0, 1, 0) z (0, 0, 1) at (0, 0, 0) in component "TAPA"
hidden bodies 2 3 1 7
